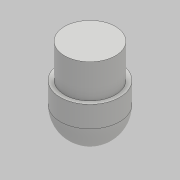
# Autodesk Inventor part: exercise2-3
Saved by Autodesk Inventor 2018 (Build 220112000, 112)
## iProperties
Created: 2020-09-19
Part Number: exercise2-3
Material: 一般
Document SubType Name: Modeling
Designer: 王鼎鈞
Density: 1 g/cm^3
Appearance: 預設
Author: 王鼎鈞
Autodesk Inventor part; units mm, degrees
ref_plane "YZ Plane" through (0, 0, 0) normal (1, 0, 0) x (0, 1, 0)
ref_plane "XZ Plane" through (0, 0, 0) normal (0, 1, 0) x (-1, 0, 0)
ref_plane "XY Plane" through (0, 0, 0) normal (0, 0, 1) x (1, 0, 0)
sketch "草圖1" plane through (0, 0, 0) normal (1, 0, 0) x (0, 1, 0)
  line L0 (-4.2249, 0) -> (25.3492, 0) projected
  line L1 (0, -64.3492) -> (0, 10.7249) projected
  line L2 (0, 0) -> (15, 0)
  line L3 (15, 0) -> (15, -20)
  line L4 (15, -20) -> (0, -20)
  line L5 (0, -20) -> (0, 0)
  line L6 (0, -20) -> (17.5, -20)
  line L7 (17.5, -20) -> (17.5, -32.5)
  line L8 (17.5, -32.5) -> (0, -32.5)
  line L9 (0, -32.5) -> (0, -20)
  arc A0 (0, -50) -> (17.5, -32.5) centre (0, -32.5) ccw
  line L10 (0, -50) -> (0, -33.1775)
  line L11 (0, -33.1775) -> (0, -32.5)
  line L12 (0, -32.5) -> (17.5, -32.5)
  dimension "d0" = 15
  dimension "d1" = 20
  dimension "d2" = 17.5
  dimension "d3" = 12.5
  constraints: 22 end point, 4 parallel, 2 collinear, 2 horizontal, 2 perpendicular, 2 point on circle, 2 point on line, 1 centre point, 1 coincident
  measures "d0" distance of L3.end L4.end
  measures "d1" distance of L2.end L3.end
  measures "d2" distance of L7.end L8.end
  measures "d3" distance of L6.end L7.end
revolve "迴轉1" add sketch "草圖1" angle 360 about axis through (0, 0, -32.5) along (0, 0, 1)
